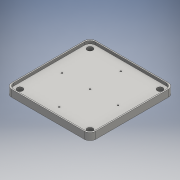
# Autodesk Inventor part: sampleHolderXYstageBase
Saved by Autodesk Inventor 2016 (Build 200138000, 138)
## iProperties
Created: 2016-11-09
Part Number: sampleHolderXYstageBase
Material: Generic
Document SubType Name: Modeling
Designer: sims01
Density: 1 g/cm^3
Appearance: Default
Author: sims01
Autodesk Inventor part; units mm, degrees
ref_plane "YZ Plane" through (0, 0, 0) normal (1, 0, 0) x (0, 1, 0)
ref_plane "XZ Plane" through (0, 0, 0) normal (0, 1, 0) x (-1, 0, 0)
ref_plane "XY Plane" through (0, 0, 0) normal (0, 0, 1) x (1, 0, 0)
sketch "Sketch5" plane through (0, 0, 0) normal (0, 0, 1) x (1, 0, 0)
  line L0 (-65, 75) -> (65, 75)
  line L1 (75, 65) -> (75, -65)
  line L2 (65, -75) -> (-65, -75)
  line L3 (-75, -65) -> (-75, 65)
  arc A0 (-65, 75) -> (-75, 65) centre (-65, 65) ccw
  arc A1 (-75, -65) -> (-65, -75) centre (-65, -65) ccw
  arc A2 (65, -75) -> (75, -65) centre (65, -65) ccw
  arc A3 (75, 65) -> (65, 75) centre (65, 65) ccw
  point P0 (0, 0)
  point P1 (-75, 75)
  point P2 (75, -75)
  point P3 (75, 75)
  dimension "d36" = 150
  dimension "d37" = 150
  dimension "d38" = 75
  dimension "d39" = 75
  dimension "d40" = 10
  constraints: 8 end point, 8 point on circle, 8 tangent, 6 point on line, 4 centre point, 3 equal radius, 2 parallel, 1 horizontal, 1 perpendicular
  measures "d36" distance of point (-75, 75) point (75, 75)
  measures "d37" distance of point (75, 75) point (75, -75)
  measures "d38" distance from line of point (0, 0) L0
  measures "d39" distance from line of point (0, 0) L1
  measures "d40" radius of A0
extrude "base" add sketch "Sketch5" along normal blind 7.5
sketch "Sketch6" plane through (0, 0, 7.5) normal (0, 0, 1) x (1, 0, 0)
  point P0 (0, 0)
  point P1 (-62.5, 62.5)
  point P2 (62.5, 62.5)
  point P3 (-62.5, -62.5)
  point P4 (62.5, -62.5)
  dimension "d43" = 125
  dimension "d44" = 125
  dimension "d45" = 62.5
  dimension "d46" = 62.5
  constraints: 2 horizontal alignment, 2 vertical alignment
  measures "d43" distance of point (62.5, 62.5) point (-62.5, 62.5)
  measures "d44" distance of point (-62.5, -62.5) point (-62.5, 62.5)
  measures "d45" horizontal distance of point (62.5, 62.5) point (0, 0)
  measures "d46" horizontal distance of point (0, 0) point (-62.5, 62.5)
hole "mountingHoles" at (-62.5, 62.5, 7.5) at (62.5, 62.5, 7.5) at (-62.5, -62.5, 7.5) at (62.5, -62.5, 7.5) direction (0, 0, -1) diameter 6.6 depth 8 tip angle 118 counterbore diameter 10 counterbore depth 6.5 clearance for "Hex Head Cap Screw ISO 24017" size "M6" standard "ISO"
sketch "Sketch7" plane through (0, 0, 7.5) normal (0, 0, 1) x (1, 0, 0)
  line L0 (-63, 73) -> (63, 73)
  line L1 (73, 63) -> (73, -63)
  line L2 (63, -73) -> (-63, -73)
  line L3 (-73, -63) -> (-73, 63)
  line L4 (65, 75) -> (-65, 75) projected
  line L5 (75, -65) -> (75, 65) projected
  line L6 (-65, -75) -> (65, -75) projected
  line L7 (-75, 65) -> (-75, -65) projected
  arc A0 (-63, 73) -> (-73, 63) centre (-63, 63) ccw
  arc A1 (-73, -63) -> (-63, -73) centre (-63, -63) ccw
  arc A2 (63, -73) -> (73, -63) centre (63, -63) ccw
  arc A3 (73, 63) -> (63, 73) centre (63, 63) ccw
  line L8 (-65, 75) -> (65, 75)
  line L9 (75, 65) -> (75, -65)
  line L10 (65, -75) -> (-65, -75)
  line L11 (-75, -65) -> (-75, 65)
  line L12 (-65, -75) -> (65, -75) projected
  arc A4 (-65, 75) -> (-75, 65) centre (-65, 65) ccw
  arc A5 (-75, -65) -> (-65, -75) centre (-65, -65) ccw
  arc A6 (65, -75) -> (75, -65) centre (65, -65) ccw
  arc A7 (75, 65) -> (65, 75) centre (65, 65) ccw
  point P0 (0, 0)
  dimension "d54" = 2
  dimension "d55" = 2
  dimension "d56" = 2
  dimension "d57" = 2
  dimension "d58" = 10
  dimension "d59" = 10
  dimension "d60" = 10
  dimension "d61" = 10
  constraints: 16 end point, 16 point on circle, 16 tangent, 8 centre point, 4 collinear, 4 equal radius, 4 parallel, 2 horizontal, 2 perpendicular
  measures "d54" distance between parallel lines of L4 L0
  measures "d55" distance between parallel lines of L5 L1
  measures "d56" distance between parallel lines of L6 L2
  measures "d57" distance between parallel lines of L7 L3
  measures "d58" radius of A0
  measures "d59" radius of A4
  measures "d60" radius of A6
  measures "d61" radius of A7
extrude "spillTray" add sketch "Sketch7" along normal blind 5
sketch "Sketch9" plane through (0, 0, 7.5) normal (0, 0, 1) x (1, 0, 0)
  circle A0 centre (0, 55) radius 1.325
  circle A1 centre (-50, 0) radius 1.325
  circle A2 centre (0, -55) radius 1.325
  circle A3 centre (50, 0) radius 1.325
  circle A4 centre (0, 0) radius 1.325
  dimension "d73" = 2.65
  dimension "d74" = 2.65
  dimension "d75" = 2.65
  dimension "d76" = 2.65
  dimension "d77" = 2.65
  dimension "d78" = 55
  dimension "d79" = 55
  dimension "d80" = 50
  dimension "d81" = 50
  constraints: 5 centre point, 2 coincident, 2 horizontal alignment, 2 vertical alignment
  measures "d73" diameter of A0
  measures "d74" diameter of A4
  measures "d75" diameter of A1
  measures "d76" diameter of A2
  measures "d77" diameter of A3
  measures "d78" distance of point (0, 0) A0.centre
  measures "d79" distance of A2.centre point (0, 0)
  measures "d80" distance of A1.centre point (0, 0)
  measures "d81" distance of A3.centre point (0, 0)
extrude "Extrusion5" cut sketch "Sketch9" against normal blind 2
equation "\"d38\" = 0.5 * d37"
equation "\"d39\" = 0.5 * d36"
equation "\"d44\" = d43"
equation "\"d45\" = 0.5 * d43"
equation "\"d46\" = 0.5 * d44"
equation "\"d55\" = d54"
equation "\"d56\" = d54"
equation "\"d57\" = d54"
equation "\"d74\" = d73"
equation "\"d75\" = d73"
equation "\"d76\" = d73"
equation "\"d77\" = d73"
equation "\"d79\" = d78"
equation "\"d81\" = d80"
body "Solid2"
